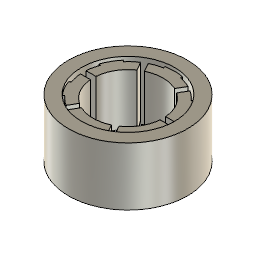
Circular Resonant Cavity v1 (Autodesk Fusion 360 design; units mm, degrees)
Autodesk Fusion 360 part; units mm, degrees
note: some values were not read from the file. Chosen so that the rebuilt part matches the saved one: which bodies a step acts on.
sketch "Sketch1" plane through (0, 0, 0) normal (0, 0, 1) x (1, 0, 0) in component "6 Electrodes"
  circle A0 centre (0, 0) radius 13.5
  circle A1 centre (0, 0) radius 18
  circle A2 centre (0, 0) radius 17.3
  circle A3 centre (0, 0) radius 23
  line L0 (13.4576, -1.069) -> (17.2669, -1.069)
  line L1 (13.4576, 1.069) -> (17.2669, 1.069)
  line L2 (7.6546, 11.1201) -> (9.5593, 14.4191)
  line L3 (5.803, 12.1891) -> (7.7077, 15.4881)
  line L4 (-5.803, 12.1891) -> (-7.7077, 15.4881)
  line L5 (-7.6546, 11.1201) -> (-9.5593, 14.4191)
  line L6 (-13.4576, 1.069) -> (-17.2669, 1.069)
  line L7 (-13.4576, -1.069) -> (-17.2669, -1.069)
  line L8 (-7.6546, -11.1201) -> (-9.5593, -14.4191)
  line L9 (-5.803, -12.1891) -> (-7.7077, -15.4881)
  line L10 (5.803, -12.1891) -> (7.7077, -15.4881)
  line L11 (7.6546, -11.1201) -> (9.5593, -14.4191)
  line L12 (3.4346, -17.6693) -> (3.301, -16.9822)
  line L13 (-3.4346, -17.6693) -> (-3.301, -16.9822)
  line L14 (17.0193, -5.8602) -> (16.3575, -5.6323)
  line L15 (13.5848, -11.8091) -> (13.0565, -11.3498)
  line L16 (13.5848, 11.8091) -> (13.0565, 11.3498)
  line L17 (17.0193, 5.8602) -> (16.3575, 5.6323)
  line L18 (-3.4346, 17.6693) -> (-3.301, 16.9822)
  line L19 (3.4346, 17.6693) -> (3.301, 16.9822)
  line L20 (-17.0193, 5.8602) -> (-16.3575, 5.6323)
  line L21 (-13.5848, 11.8091) -> (-13.0565, 11.3498)
  line L22 (-13.5848, -11.8091) -> (-13.0565, -11.3498)
  line L23 (-17.0193, -5.8602) -> (-16.3575, -5.6323)
  dimension "d51" = 1.069
  dimension "d52" = 1.069
  dimension "d54" = 360
  dimension "d56" = 360
  constraint coincident A0 L0.start
  constraint coincident A2 L0.end
  constraint coincident A1 L12.start
  constraint coincident A2 L12.end
  constraint coincident A1 L13.start
  constraint coincident A2 L13.end
  measures "d51" vertical distance of A0.centre L0.start
  measures "d52" vertical distance of A0.centre L0.end
extrude "Extrude1" add sketch "Sketch1" along normal mid plane 20 contours A0 A2 L1 L2 | A0 A2 L0 L11 | A0 A2 L3 L4 | A1 A2 L16 L17 | A0 A2 L9 L10 | A1 A2 L14 L15 | A0 A2 L5 L6 | A1 A2 L18 L19 | A0 A2 L7 L8 | A1 A2 L12 L13 | A1 A2 L20 L21 | A1 A2 L22 L23 makes body 1 at (-2.6487, 13.2376, 3.3333) makes body 2 at (13.3885, -1.7318, 3.3333) makes body 3 at (-8.7135, 10.3114, 3.3333) makes body 4 at (12.2998, 5.5646, 3.3333) makes body 5 at (5.1944, -12.4607, 3.3333) makes body 6 at (-10.969, -7.8697, 3.3333) in component "6 Electrodes"
extrude "Extrude2" add sketch "Sketch1" along normal mid plane 22.5 bodies 1 2 3 4 5 6 in component "6 Electrodes"
sketch "Sketch1 (2)" plane through (0, 0, 0) normal (0, 0, 1) x (1, 0, 0) in component "4 Electrodes"
  circle A0 centre (0, 0) radius 7.5
  circle A1 centre (0, 0) radius 10.2
  circle A2 centre (0, 0) radius 9.3
  circle A3 centre (0, 0) radius 15.2
  line L0 (7.4882, -0.4205) -> (9.2905, -0.4205)
  line L1 (7.4882, 0.4205) -> (9.2905, 0.4205)
  line L2 (0.4205, 7.4882) -> (0.4205, 9.2905)
  line L3 (-0.4205, 7.4882) -> (-0.4205, 9.2905)
  line L4 (-7.4882, 0.4205) -> (-9.2905, 0.4205)
  line L5 (-7.4882, -0.4205) -> (-9.2905, -0.4205)
  line L6 (-0.4205, -7.4882) -> (-0.4205, -9.2905)
  line L7 (0.4205, -7.4882) -> (0.4205, -9.2905)
  line L8 (-4.4714, -9.1677) -> (-4.0769, -8.3588)
  line L9 (-9.1677, -4.4714) -> (-8.3588, -4.0769)
  line L10 (9.1677, -4.4714) -> (8.3588, -4.0769)
  line L11 (4.4714, -9.1677) -> (4.0769, -8.3588)
  line L12 (4.4714, 9.1677) -> (4.0769, 8.3588)
  line L13 (9.1677, 4.4714) -> (8.3588, 4.0769)
  line L14 (-9.1677, 4.4714) -> (-8.3588, 4.0769)
  line L15 (-4.4714, 9.1677) -> (-4.0769, 8.3588)
  dimension "d61" = 0.4205
  dimension "d62" = 0.4205
  dimension "d64" = 360
  dimension "d66" = 360
  constraint coincident A0 L0.start
  constraint coincident A2 L0.end
  constraint coincident A1 L8.start
  constraint coincident A2 L8.end
  constraint coincident A1 L9.start
  constraint coincident A2 L9.end
  measures "d61" vertical distance of A0.centre L0.start
  measures "d62" vertical distance of A0.centre L0.end
extrude "Extrude1'" add sketch "Sketch1 (2)" along normal mid plane 15 separate body contours A0 A2 L1 L2 | A0 A2 L0 L7 | A0 A2 L3 L4 | A1 A2 L12 L13 | A0 A2 L5 L6 | A1 A2 L10 L11 | A1 A2 L14 L15 | A1 A2 L8 L9 makes body 7 at (-7.412, 1.1455, 2.5) makes body 8 at (5.5548, -5.0393, 2.5) makes body 9 at (3.8708, 6.4239, 2.5) makes body 10 at (-3.2288, -6.7694, -2.5) in component "4 Electrodes"
extrude "Extrude2'" add sketch "Sketch1 (2)" along normal mid plane 17.5 bodies 7 8 9 10 in component "4 Electrodes"
component "6 Electrodes" placed x (1, 0, 0) y (0, 1, 0) z (0, 0, 1) at (0, 0, 0)
component "4 Electrodes" placed x (1, 0, 0) y (0, 1, 0) z (0, 0, 1) at (0, 0, 0)
